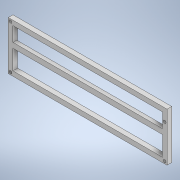
# Autodesk Inventor part: lateral suport
Saved by Autodesk Inventor 2021.2 (Build 252289000, 289)
## iProperties
Created: 2024-04-24
Part Number: lateral suport
Material: Generic
Document SubType Name: Modeling
Designer: cioba
Density: 1 g/cm^3
Appearance: Default
Author: cioba
Autodesk Inventor part; units mm, degrees
ref_plane "YZ Plane" through (0, 0, 0) normal (1, 0, 0) x (0, 1, 0)
ref_plane "XZ Plane" through (0, 0, 0) normal (0, 1, 0) x (-1, 0, 0)
sketch "Sketch1" plane through (0, 0, 0) normal (0, 0, 1) x (1, 0, 0)
  line L0 (-201.7062, 85.6066) -> (-31.7062, 85.6066)
  line L1 (-31.7062, 85.6066) -> (-31.7062, 33.6066)
  line L2 (-31.7062, 33.6066) -> (-201.7062, 33.6066)
  line L3 (-201.7062, 33.6066) -> (-201.7062, 85.6066)
  line L4 (-36.7062, 80.6066) -> (-196.7062, 80.6066)
  line L5 (-196.7062, 38.6066) -> (-36.7062, 38.6066)
  line L6 (-196.7062, 59.6066) -> (-36.7062, 59.6066)
  line L7 (-36.7062, 65.0934) -> (-196.7062, 65.0934)
  line L8 (-36.7062, 38.6066) -> (-36.7062, 59.6066)
  line L9 (-36.7062, 65.0934) -> (-36.7062, 80.6066)
  line L10 (-196.7062, 80.6066) -> (-196.7062, 65.0934)
  line L11 (-196.7062, 59.6066) -> (-196.7062, 38.6066)
  line L12 (-196.7062, 80.6066) -> (-201.7062, 80.6066)
  line L13 (-36.7062, 80.6066) -> (-31.7062, 80.6066)
  line L14 (-36.7062, 80.6066) -> (-36.7062, 85.6066)
  line L15 (-36.7062, 38.6066) -> (-36.7062, 33.6066)
  line L16 (-36.7062, 38.6066) -> (-31.7062, 38.6066)
  line L17 (-196.7062, 38.6066) -> (-201.7062, 38.6066)
  line L18 (-196.7062, 38.6066) -> (-196.7062, 33.6066)
  line L19 (-196.7062, 80.6066) -> (-196.7062, 85.6066)
  circle A0 centre (-199.2062, 83.1066) radius 2.5
  circle A1 centre (-199.2062, 36.1066) radius 2.5
  circle A2 centre (-34.2062, 36.1066) radius 2.5
  circle A3 centre (-34.2062, 72.6066) radius 2.5
  point P0 (0, 0)
  constraints: 40 end point, 11 point on line, 9 perpendicular, 7 parallel, 4 centre point, 1 horizontal, 1 tangent, 1 vertical
extrude "Extrusion1" add sketch "Sketch1" against normal blind 5 contours L19 A0 L0 | L0 L14 L4 L19 | L0 L1 L13 L14 | A0 L3 L0 | A0 | L19 L12 A0 | L13 L1 A3 L9 | A0 L12 L3 | L10 L7 L9 A3 L1 L16 L8 L6 L11 L17 L3 L12 | A3 | L17 A1 L3 | L1 A2 L16 | A1 L2 L3 | A1 | L17 L18 A1 | A2 | L1 L2 A2 | A2 L15 L16 | A1 L18 L2 | L5 L15 L2 L18 | L2 L15 A2
ref_plane "Work Plane1" through (-31.7062, 85.6066, -5) normal (0, 0, 1) x (1, 0, 0)
sketch "Sketch2" plane through (0, 0, -5) normal (0, 0, -1) x (-1, 0, 0)
  line L0 (36.7062, 65.0934) -> (196.7062, 65.0934)
  line L1 (196.7062, 65.0934) -> (196.7062, 59.6066)
  line L2 (196.7062, 59.6066) -> (36.7062, 59.6066)
  line L3 (36.7062, 59.6066) -> (36.7062, 65.0934)
  point P0 (0, 0)
  constraints: 8 end point, 2 parallel, 1 horizontal, 1 perpendicular
extrude "Extrusion2" cut sketch "Sketch2" against normal blind 1
hole "Hole1" at (-199.2062, 83.1066, 0) direction (0, 0, -1) diameter 3 depth 5 tip angle 118
hole "Hole2" at (-199.2062, 36.1066, 0) direction (0, 0, -1) diameter 3 depth 5 tip angle 118
hole "Hole4" at (-34.2062, 36.1066, 0) direction (0, 0, -1) diameter 3 depth 5 tip angle 118
hole "Hole5" at (-34.2062, 72.6066, 0) direction (0, 0, -1) diameter 3 depth 5 tip angle 118
thread "Thread1" size "M3x0.5" class "6H" standard "ANSI Metric M Profile" full length
thread "Thread2" size "M3x0.5" class "6H" standard "ANSI Metric M Profile" full length
thread "Thread3" size "M3x0.5" class "6H" standard "ANSI Metric M Profile" full length
thread "Thread4" size "M3x0.5" class "6H" standard "ANSI Metric M Profile" full length
body "Solid1"
